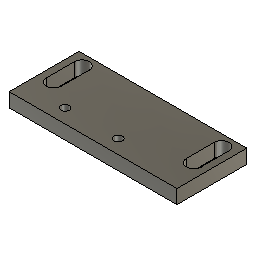
Mechanical Endstop Mount (Autodesk Fusion 360 design; units mm, degrees)
Autodesk Fusion 360 part; units mm, degrees
sketch "Sketch1" plane through (0, 0, 0) normal (0, 0, 1) x (1, 0, 0)
  line L0 (30, -12.5) -> (-30, -12.5)
  line L1 (-30, -12.5) -> (-30, 12.5)
  line L2 (-30, 12.5) -> (30, 12.5)
  line L3 (30, 12.5) -> (30, -12.5)
  line L4 (30, -12.5) -> (-30, 12.5) construction
  line L5 (-30, -12.5) -> (30, 12.5) construction
  circle A0 centre (-15, -7.5) radius 1.5
  circle A1 centre (4, -7.5) radius 1.5
  line L6 (-27.625, 8.5) -> (-27.625, -1.5)
  arc A2 (-27.625, -1.5) -> (-22.375, -1.5) centre (-25, -1.5) ccw
  line L7 (-22.375, -1.5) -> (-22.375, 8.5)
  arc A3 (-22.375, 8.5) -> (-27.625, 8.5) centre (-25, 8.5) ccw
  line L8 (-25, 8.5) -> (-25, -1.5) construction
  line L9 (27.625, -1.5) -> (27.625, 8.5)
  arc A4 (27.625, 8.5) -> (22.375, 8.5) centre (25, 8.5) ccw
  line L10 (22.375, 8.5) -> (22.375, -1.5)
  arc A5 (22.375, -1.5) -> (27.625, -1.5) centre (25, -1.5) ccw
  line L11 (25, -1.5) -> (25, 8.5) construction
  dimension "d1" = 60
  dimension "d2" = 25
  dimension "d3" = 3
  dimension "d4" = 3
  dimension "d5" = 19
  dimension "d6" = 5
  dimension "d7" = 5
  dimension "d8" = 15
  dimension "d9" = 5.25
  dimension "d10" = 5.25
  dimension "d11" = 5
  dimension "d12" = 5
  dimension "d15" = 4
  dimension "d16" = 4
  dimension "d17" = 10
  dimension "d18" = 10
  constraint horizontal L0
  constraint perpendicular L0 L1
  constraint parallel L0 L2
  constraint parallel L1 L3
  constraint coincident L4 origin
  constraint coincident L5 origin
  constraint tangent L6 A2
  constraint tangent A2 L7
  constraint parallel L6 L7
  constraint tangent L7 A3
  constraint tangent L6 A3
  constraint vertical L8
  constraint tangent L9 A4
  constraint tangent A4 L10
  constraint parallel L9 L10
  constraint tangent L10 A5
  constraint tangent L9 A5
  constraint vertical L11
  measures "d1" distance of L1.end L2.end
  measures "d2" distance of L0.end L1.end
  measures "d3" diameter of A0
  measures "d4" diameter of A1
  measures "d5" distance of A0.centre A1.centre
  measures "d6" distance of L0 A0.centre
  measures "d7" distance of L0 A1.centre
  measures "d8" distance of L1 A0.centre
  measures "d9" diameter of A2
  measures "d10" diameter of A4
  measures "d11" distance of L1 A2.centre
  measures "d12" distance of L3 A4.centre
  measures "d15" distance of L2 A3.centre
  measures "d16" distance of L2 A4.centre
  measures "d17" distance of A3.centre A2.centre
  measures "d18" distance of A5.centre A4.centre
extrude "Extrude1" add sketch "Sketch1" along normal blind 5
equation "d7 = d6"
equation "d10 = d9"
equation "d12 = d11"
equation "d16 = d15"
equation "d18 = d17"
